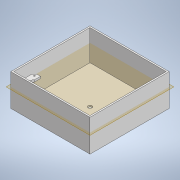
# Autodesk Inventor part: Base
Saved by Autodesk Inventor 2022 (Build 260153000, 153)
## iProperties
Created: 2022-02-27
Part Number: Base
Material: Generic
Document SubType Name: Modeling
Designer: alexo
Density: 1 g/cm^3
Appearance: Default
Author: alexo
Autodesk Inventor part; units mm, degrees
ref_plane "YZ Plane" through (0, 0, 0) normal (1, 0, 0) x (0, 1, 0)
ref_plane "XZ Plane" through (0, 0, 0) normal (0, 1, 0) x (-1, 0, 0)
sketch "Sketch1" plane through (0, 0, 0) normal (0, 1, 0) x (-1, 0, 0)
  line L0 (-80.6, -80.6) -> (80.6, -80.6)
  line L1 (80.6, -80.6) -> (80.6, 80.6)
  line L2 (80.6, 80.6) -> (-80.6, 80.6)
  line L3 (-80.6, 80.6) -> (-80.6, -80.6)
  line L4 (-80.6, -80.6) -> (80.6, 80.6) construction
  line L5 (80.6, -80.6) -> (-80.6, 80.6) construction
  point P0 (0, 0)
  dimension "d0" = 161.2
  constraints: 12 end point, 2 midpoint, 2 parallel, 2 perpendicular, 1 horizontal
  measures "d0" distance of L0.end L1.end
extrude "Extrusion1" add sketch "Sketch1" along normal blind 3
sketch "Sketch2" plane through (0, 3, 0) normal (0, 1, 0) x (1, 0, 0)
  line L0 (-80.6, 80.6) -> (-80.6, -80.6) projected
  line L1 (-80.6, -80.6) -> (80.6, -80.6) projected
  line L2 (80.6, -80.6) -> (80.6, 80.6) projected
  line L3 (80.6, 80.6) -> (-80.6, 80.6) projected
  line L4 (77.6, 77.6) -> (-77.6, 77.6)
  line L5 (-77.6, 77.6) -> (-77.6, -77.6)
  line L6 (-77.6, -77.6) -> (77.6, -77.6)
  line L7 (77.6, -77.6) -> (77.6, 77.6)
  line L8 (77.6, 77.6) -> (-77.6, -77.6) construction
  line L9 (-77.6, 77.6) -> (77.6, -77.6) construction
  point P0 (0, 0)
  dimension "d3" = 3
  dimension "d4" = 3
  constraints: 12 end point, 2 midpoint, 2 parallel, 1 horizontal, 1 perpendicular
  measures "d3" distance between parallel lines of L0 L5
  measures "d4" distance between parallel lines of L1 L6
extrude "Extrusion2" add sketch "Sketch2" along normal blind 62
sketch "Sketch3" plane through (0, 3, 0) normal (0, 1, 0) x (1, 0, 0)
  circle A0 centre (0, 0) radius 14
  dimension "d7" = 28
  constraints: 1 centre point, 1 coincident
  measures "d7" diameter of A0
extrude "Extrusion3" cut sketch "Sketch3" against normal blind 44.5
ref_plane "Work Plane1" through (0, 38, 0) normal (0, 1, 0) x (1, 0, 0)
sketch "Sketch4" plane through (0, 38, 0) normal (0, 1, 0) x (1, 0, 0)
  line L0 (-77.6, -40.6) -> (-77.6, -72.6) projected
  line L1 (-77.6, -72.6) -> (-72.6, -77.6) construction
  line L2 (-72.6, -77.6) -> (-40.6, -77.6) projected
  line L3 (-40.6, -77.6) -> (-35.6, -72.6) construction
  line L4 (-35.6, -72.6) -> (-35.6, -40.6) projected
  line L5 (-35.6, -40.6) -> (-40.6, -35.6) projected
  line L6 (-40.6, -35.6) -> (-72.6, -35.6) projected
  line L7 (-72.6, -35.6) -> (-77.6, -40.6) construction
  circle A0 centre (-72.1, -41.1) radius 1.5 projected
  circle A1 centre (-72.1, -72.1) radius 1.5 projected
  circle A2 centre (-41.1, -72.1) radius 1.5 projected
  circle A3 centre (-41.1, -41.1) radius 1.5 projected
  circle A4 centre (-56.6, -56.6) radius 11 construction
  line L8 (-38.1, -75.1) -> (-75.1, -38.1) construction
  arc A5 (-65.0853, -48.1147) -> (-48.1147, -65.0853) centre (-56.6, -56.6) ccw
  arc A6 (-48.1147, -65.0853) -> (-65.0853, -48.1147) centre (-56.6, -56.6) ccw construction
  line L9 (-65.0853, -48.1147) -> (-65.0853, -35.6)
  line L10 (-48.1147, -65.0853) -> (-35.6, -65.0853)
  line L11 (-77.6, -77.6) -> (-77.6, 77.6) projected
  line L12 (77.6, -77.6) -> (-77.6, -77.6) projected
  line L13 (-35.6, -72.6) -> (-35.6, -77.6)
  line L14 (-72.6, -35.6) -> (-77.6, -35.6)
  point P0 (0, 0)
  dimension "d11" = 24
  constraints: 10 end point, 6 point on line, 4 perpendicular, 4 point on circle, 2 centre point, 2 midpoint, 1 coincident
  measures "d11" diameter of A5
extrude "Extrusion4" add sketch "Sketch4" along normal blind 4 contours L11 L14 L6 L9 A5 L10 L4 L13 L12 L2 L0
sketch "Sketch5" plane through (0, 3, 0) normal (0, 1, 0) x (1, 0, 0)
  circle A0 centre (0, 0) radius 14 projected
  line L0 (77.6, 77.6) -> (-77.6, 77.6) projected
  line L1 (-77.6, 77.6) -> (-77.6, -77.6) projected
  line L2 (-77.6, -77.6) -> (77.6, -77.6) projected
  line L3 (77.6, -77.6) -> (77.6, 77.6) projected
  circle A1 centre (0, 0) radius 17
  dimension "d14" = 3
  constraints: 1 centre point, 1 coincident
  measures "d14" radial gap between concentric circles of A0 A1
ref_plane "Work Plane2" through (-5.2503, 8.15, -5.2503) normal (0, 1, 0) x (-0.7071, 0, 0.7071)
extrude "Extrusion5" add sketch "Sketch5" along normal up to surface (5.15 mm away) contours A1
sketch "Sketch6" plane through (0, 8.15, 0) normal (0, 1, 0) x (1, 0, 0)
  circle A0 centre (0, 0) radius 17 projected
  circle A1 centre (0, 0) radius 8
  point P0 (0, 0)
  dimension "d17" = 16
  constraints: 1 centre point, 1 coincident
  measures "d17" diameter of A1
extrude "Extrusion6" add sketch "Sketch6" along normal blind 5
sketch "Sketch7" plane through (0, 13.15, 0) normal (0, 1, 0) x (1, 0, 0)
  circle A0 centre (0, 0) radius 17 projected
  circle A1 centre (0, 0) radius 3
  point P0 (0, 0)
  dimension "d20" = 6
  constraints: 1 centre point, 1 coincident
  measures "d20" diameter of A1
extrude "Extrusion7" add sketch "Sketch7" along normal blind 24
sketch "Sketch9" plane through (0, 37.15, 0) normal (0, 1, 0) x (1, 0, 0)
  circle A0 centre (0, 0) radius 8
  circle A1 centre (0, 0) radius 17 projected
  point P0 (0, 0)
  dimension "d23" = 16
  constraints: 1 centre point, 1 coincident
  measures "d23" diameter of A0
extrude "Extrusion8" add sketch "Sketch9" along normal blind 5
equation "\"d0\" = Lenght"
equation "\"d1\" = Gr"
equation "\"d3\" = Gr"
equation "\"d4\" = Gr"
equation "\"d14\" = Gr"
equation "\"d17\" = bearing"
equation "\"d23\" = bearing"
equation "\"Gr\" = 3"
equation "\"Lenght\" = 161.2"
equation "\"bearing\" = 16"
body "Solid1"
